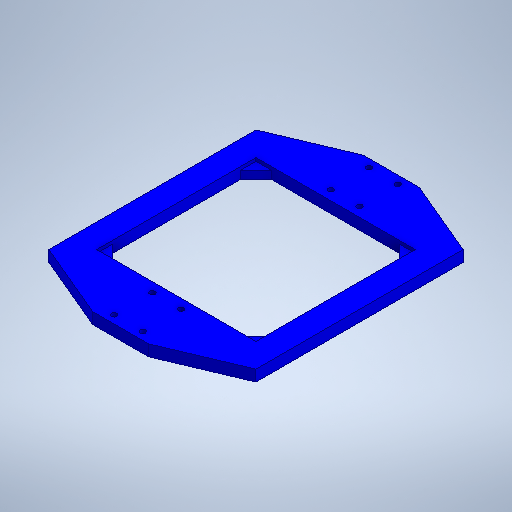
# Autodesk Inventor part: BedHousingFrame
Saved by Autodesk Inventor 2025.2 (Build 292293000, 293)
## iProperties
Created: 2025-05-31
Part Number: BedHousingFrame
Material: Generic
Document SubType Name: Modeling
Designer: Simon
Density: 1 g/cm^3
Appearance: Default(2)
Author: Simon
Autodesk Inventor part; units mm, degrees
ref_plane "YZ Plane" through (0, 0, 0) normal (1, 0, 0) x (0, 1, 0)
ref_plane "XZ Plane" through (0, 0, 0) normal (0, 1, 0) x (-1, 0, 0)
ref_plane "XY Plane" through (0, 0, 0) normal (0, 0, 1) x (1, 0, 0)
sketch "Sketch1" plane through (0, 0, 0) normal (0, 1, 0) x (-1, 0, 0)
  line L0 (0, 0) -> (100, 0)
  line L1 (100, 0) -> (100, -100)
  line L2 (100, -100) -> (0, -100)
  line L3 (0, -100) -> (0, 0)
  line L4 (100, 0) -> (0, -100)
  line L5 (100, -100) -> (0, 0)
  line L6 (-15, 35) -> (115, 35)
  line L7 (115, 35) -> (115, -135)
  line L8 (115, -135) -> (-15, -135)
  line L9 (-15, -135) -> (-15, 35)
  line L10 (-15, 35) -> (115, -135) construction
  line L11 (115, 35) -> (-15, -135) construction
  line L12 (115, 35) -> (115, 15)
  line L13 (115, 15) -> (75, 15)
  line L14 (75, 15) -> (75, 35)
  line L15 (-15, 35) -> (-15, 15)
  line L16 (-15, 15) -> (25, 15)
  line L17 (25, 15) -> (25, 35)
  line L18 (75, 15) -> (67.5, 15)
  line L19 (67.5, 15) -> (67.5, 35)
  line L20 (25, 15) -> (32.5, 15)
  line L21 (32.5, 15) -> (32.5, 35)
  line L22 (32.5, 35) -> (-15, 15)
  line L23 (67.5, 35) -> (115, 15)
  line L24 (115, -135) -> (115, -115)
  line L25 (115, -115) -> (67.5, -115)
  line L26 (67.5, -115) -> (67.5, -135)
  line L27 (-15, -135) -> (-15, -115)
  line L28 (-15, -115) -> (32.5, -115)
  line L29 (32.5, -115) -> (32.5, -135)
  line L30 (115, -115) -> (67.5, -135)
  line L31 (-15, -115) -> (32.5, -135)
  line L32 (100, 0) -> (100, -10)
  line L33 (100, -10) -> (90, -10)
  line L34 (90, -10) -> (90, 0)
  line L35 (100, -100) -> (100, -90)
  line L36 (100, -90) -> (90, -90)
  line L37 (90, -90) -> (90, -100)
  line L38 (0, -100) -> (10, -100)
  line L39 (10, -100) -> (10, -90)
  line L40 (10, -90) -> (0, -90)
  line L41 (0, 0) -> (10, 0)
  line L42 (10, 0) -> (10, -10)
  line L43 (0, -10) -> (10, -10)
  line L44 (90, 0) -> (100, -10)
  line L45 (100, -90) -> (90, -100)
  line L46 (0, -90) -> (10, -100)
  line L47 (10, 0) -> (0, -10)
  line L48 (50, -135) -> (50, -130)
  line L49 (41, -130) -> (59, -130)
  line L50 (59, -130) -> (59, -106)
  line L51 (59, -106) -> (41, -106)
  line L52 (41, -106) -> (41, -130)
  line L53 (50, 35) -> (50, 30)
  line L54 (41, 30) -> (59, 30)
  line L55 (59, 30) -> (59, 6)
  line L56 (59, 6) -> (41, 6)
  line L57 (41, 6) -> (41, 30)
  point P0 (50, -50)
  dimension "d0" = 100
  dimension "d1" = 100
  dimension "d4" = 130
  dimension "d5" = 170
  dimension "d6" = 20
  dimension "d7" = 40
  dimension "d8" = 40
  dimension "d10" = 7.5
  dimension "d11" = 7.5
  dimension "d12" = 20
  dimension "d13" = 47.5
  dimension "d14" = 10
  dimension "d15" = 10
  dimension "d16" = 10
  dimension "d17" = 10
  dimension "d22" = 5
  dimension "d23" = 18
  dimension "d24" = 24
  dimension "d25" = 5
  dimension "d26" = 18
  dimension "d27" = 24
  constraints: 116 end point, 34 point on line, 17 perpendicular, 7 midpoint, 6 horizontal, 6 parallel, 2 vertical
  measures "d0" distance of L1.end L2.end
  measures "d1" distance of L0.end L1.end
  measures "d4" distance of L7.end L8.end
  measures "d5" distance of L6.end L7.end
  measures "d6" distance of L6.end L12.end
  measures "d7" distance of L13.start L13.end
  measures "d8" distance of L15.end L16.end
  measures "d10" distance of L13.end L18.end
  measures "d11" distance of L16.end L20.end
  measures "d12" distance of L7.end L24.end
  measures "d13" distance of L24.end L25.end
  measures "d14" distance of L0.end L32.end
  measures "d15" distance of L1.end L35.end
  measures "d16" distance of L2.end L38.end
  measures "d17" distance of L0.start L41.end
  measures "d22" distance of L48.start L48.end
  measures "d23" distance of L49.start L49.end
  measures "d24" distance of L49.end L50.end
  measures "d25" distance of L53.start L53.end
  measures "d26" distance of L54.start L54.end
  measures "d27" distance of L54.end L55.end
extrude "Extrusion1" add sketch "Sketch1" against normal blind 5 contours L5 L47 L3 | L0 L47 L5 | L0 L4 L44 | L46 L4 L3 | L1 L44 L4 | L4 L46 L2 | L1 L5 L45 | L5 L2 L45 | L49 L52 L51 L50 | L54 L55 L56 L57 | L16 L20 L21 L6 L19 L18 L13 L7 L25 L26 L8 L29 L28 L9 | L22 L17 L16 | L21 L20 L17 L22 | L28 L29 L31 | L23 L14 L18 L19 | L23 L13 L14 | L26 L25 L30
extrude "Extrusion2" add sketch "Sketch1" along normal blind 2 contours L49 L52 L51 L50 | L54 L55 L56 L57 | L16 L20 L21 L6 L19 L18 L13 L7 L25 L26 L8 L29 L28 L9 | L22 L17 L16 | L21 L20 L17 L22 | L28 L29 L31 | L23 L14 L18 L19 | L23 L13 L14 | L26 L25 L30
hole "Hole1" at (-59, 0, 30) at (-59, 0, 6) at (-41, 0, 30) at (-41, 0, 6) at (-59, 0, -130) at (-41, 0, -130) at (-41, 0, -106) at (-59, 0, -106) direction (0, -1, 0) diameter 3.4 end through all both
body "Solid1"
